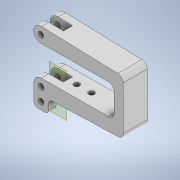
# Autodesk Inventor part: frame-1
Saved by Autodesk Inventor 2020 (Build 240168000, 168)
## iProperties
Created: 2019-10-15
Part Number: frame-1
Material: Generic
Document SubType Name: Modeling
Designer: psrob
Density: 1 g/cm^3
Appearance: Default
Author: psrob
Autodesk Inventor part; units mm, degrees
ref_plane "YZ Plane" through (0, 0, 0) normal (1, 0, 0) x (0, 1, 0)
ref_plane "XZ Plane" through (0, 0, 0) normal (0, 1, 0) x (-1, 0, 0)
ref_plane "XY Plane" through (0, 0, 0) normal (0, 0, 1) x (1, 0, 0)
sketch "Sketch1" plane through (0, 0, 0) normal (0, 0, 1) x (1, 0, 0)
  circle A0 centre (1.5, 0) radius 1.5
  circle A1 centre (1.648979, -24.25) radius 1.5
  circle A2 centre (1.648979, -31.25) radius 1.5
  circle A3 centre (1.5, 0) radius 4
  circle A4 centre (1.648979, -24.25) radius 4
  line L0 (1.5, 0) -> (33.5, 0)
  line L1 (1.648979, -24.25) -> (33.648979, -24.25)
  line L2 (33.5, 0) -> (33.648979, -24.25)
  line L3 (35.982292, 2.890075) -> (30.982386, 2.859359)
  line L4 (30.982386, 2.859359) -> (31.166687, -27.140075)
  line L5 (31.166687, -27.140075) -> (36.166593, -27.109359)
  line L6 (36.166593, -27.109359) -> (35.982292, 2.890075)
  line L7 (35.982292, 2.890075) -> (31.166687, -27.140075) construction
  line L8 (30.982386, 2.859359) -> (36.166593, -27.109359) construction
  line L9 (35.982292, 2.890075) -> (1.5, 4)
  line L10 (36.166593, -27.109359) -> (1.781342, -28.247809)
  line L11 (1.648979, -24.25) -> (1.781342, -28.247809)
  line L12 (1.516617, -20.252191) -> (31.123254, -20.070303)
  line L13 (1.5, 0) -> (1.524573, -3.999925)
  line L14 (1.524573, -3.999925) -> (31.023413, -3.818699)
  line L15 (1.5, 0) -> (1.5, 4)
  line L16 (5.648979, -24.25) -> (-2.351021, -24.25)
  line L17 (-2.351021, -24.25) -> (-2.351021, -35.25)
  line L18 (-2.351021, -35.25) -> (5.648979, -35.25)
  line L19 (5.648979, -35.25) -> (5.648979, -24.25)
  point P0 (0, 0)
  point P1 (33.57449, -12.125)
  point P2 (5.648979, -28.119757)
  point P3 (1.757239, 3.99172)
  point P4 (1.732213, -20.250866)
  dimension "d0" = 8
  dimension "d1" = 8
  dimension "d2" = 32
  dimension "d3" = 32
  dimension "d4" = 5
  dimension "d5" = 30
  dimension "d6" = 8
  dimension "d7" = 11
  constraints: 40 end point, 7 perpendicular, 5 point on circle, 4 parallel, 4 point on line, 3 horizontal, 3 midpoint, 2 centre point, 2 coincident, 1 horizontal alignment, 1 tangent, 1 vertical
  measures "d0" diameter of A3
  measures "d1" diameter of A4
  measures "d2" distance of L0.start L0.end
  measures "d3" distance of L1.start L1.end
  measures "d4" distance of L3.start L3.end
  measures "d5" distance of L4.end L3.end
  measures "d6" distance of L18.end L17.end
  measures "d7" distance of L17.end L16.end
extrude "Extrusion1" add sketch "Sketch1" along normal blind 4
sketch "Sketch2" plane through (0, 0, 4) normal (0, 0, 1) x (1, 0, 0)
  circle A0 centre (1.5, 0) radius 1.5
  circle A1 centre (1.648979, -24.25) radius 1.5
  point P0 (0, 0)
  constraints: 1 horizontal alignment
extrude "Extrusion2" cut sketch "Sketch2" against normal blind 5
fillet "Fillet1" radius 2 3 edges at (5.649, -28.1198, 2) (5.649, -35.25, 2) (-2.351, -35.25, 2)
fillet "Fillet2" radius 3 4 edges at (35.9823, 2.8901, 2) (36.1666, -27.1094, 2) (31.0234, -3.8187, 2) (31.1233, -20.0703, 2)
ref_plane "Work Plane1" through (-2.702041, -20.25, -5) normal (0, 0, -1) x (-1, 0, 0)
sketch "Sketch3" plane through (-2.702041, -20.25, -5) normal (0, 0, -1) x (-1, 0, 0)
  circle A0 centre (-4.351021, -4) radius 1.5
  circle A1 centre (-4.202041, 20.25) radius 1.5
  arc A2 (-38.850694, -3.939203) -> (-35.950022, -6.95599) centre (-35.850751, -3.957633) ccw
  line L0 (-10.284839, -7.805731) -> (-35.950022, -6.95599)
  arc A3 (-8.351021, -9.804635) -> (-10.284839, -7.805731) centre (-10.351021, -9.804635) ccw
  line L1 (-8.351021, -13) -> (-8.351021, -9.804635)
  arc A4 (-8.351021, -13) -> (-6.351021, -15) centre (-6.351021, -13) ccw
  line L2 (-2.351021, -15) -> (-6.351021, -15)
  arc A5 (-2.351021, -15) -> (-0.351021, -13) centre (-2.351021, -13) ccw
  line L3 (-0.351021, -4) -> (-0.351021, -13)
  arc A6 (-0.351021, -4) -> (-4.434254, -0.000866) centre (-4.351021, -4) ccw
  line L4 (-30.825352, 0.161267) -> (-4.434254, -0.000866)
  arc A7 (-33.806865, 3.179641) -> (-30.825352, 0.161267) centre (-30.806922, 3.161211) ccw
  line L5 (-33.743884, 13.431358) -> (-33.806865, 3.179641)
  arc A8 (-30.725511, 16.412871) -> (-33.743884, 13.431358) centre (-30.743941, 13.412928) ccw
  line L6 (-4.226615, 16.250075) -> (-30.725511, 16.412871)
  arc A9 (-4.226615, 16.250075) -> (-4.459281, 24.24172) centre (-4.202041, 20.25) ccw
  line L7 (-35.798641, 23.232961) -> (-4.459281, 24.24172)
  arc A10 (-35.798641, 23.232961) -> (-38.70207, 20.252944) centre (-35.702127, 20.234514) ccw
  line L8 (-38.850694, -3.939203) -> (-38.70207, 20.252944)
  circle A11 centre (-4.351021, -11) radius 1.5
  point P0 (-2.702041, 20.25)
extrude "Extrusion3" add sketch "Sketch3" along normal blind 4
sketch "Sketch4" plane through (0, 0, 0) normal (0, 0, -1) x (-1, 0, 0)
  arc A0 (-5.648979, -30.054635) -> (-7.582798, -28.055731) centre (-7.648979, -30.054635) ccw
  line L0 (-5.648979, -30.054635) -> (-5.648979, -33.25)
  arc A1 (-5.648979, -33.25) -> (-3.648979, -35.25) centre (-3.648979, -33.25) ccw
  line L1 (-3.648979, -35.25) -> (0.351021, -35.25)
  arc A2 (0.351021, -35.25) -> (2.351021, -33.25) centre (0.351021, -33.25) ccw
  line L2 (2.351021, -33.25) -> (2.351021, -24.25)
  arc A3 (2.351021, -24.25) -> (-1.732213, -20.250866) centre (-1.648979, -24.25) ccw
  line L3 (-1.732213, -20.250866) -> (-28.123311, -20.088733)
  arc A4 (-31.104824, -17.070359) -> (-28.123311, -20.088733) centre (-28.104881, -17.088789) ccw
  line L4 (-31.104824, -17.070359) -> (-31.041843, -6.818642)
  arc A5 (-28.02347, -3.837129) -> (-31.041843, -6.818642) centre (-28.0419, -6.837072) ccw
  line L5 (-28.02347, -3.837129) -> (-1.524573, -3.999925)
  arc A6 (-1.524573, -3.999925) -> (-1.757239, 3.99172) centre (-1.5, 0) ccw
  line L6 (-1.757239, 3.99172) -> (-33.0966, 2.982961)
  arc A7 (-33.0966, 2.982961) -> (-36.000029, 0.002944) centre (-33.000086, -0.015486) ccw
  line L7 (-36.000029, 0.002944) -> (-36.148653, -24.189203)
  arc A8 (-36.148653, -24.189203) -> (-33.247981, -27.20599) centre (-33.14871, -24.207633) ccw
  line L8 (-33.247981, -27.20599) -> (-7.582798, -28.055731)
  circle A9 centre (-1.648979, -31.25) radius 1.5
  circle A10 centre (-1.5, 0) radius 1.5
  circle A11 centre (-1.648979, -24.25) radius 1.5
  line L9 (-33.247981, -27.20599) -> (-7.582798, -28.055731)
  line L10 (-7.582798, -28.055731) -> (-7.582798, -20.214923)
  line L11 (-28.123311, -20.088733) -> (-1.732213, -20.250866)
  line L12 (-28.02347, -3.837129) -> (-1.524573, -3.999925)
  line L13 (-7.582798, -3.962706) -> (-7.582798, 3.804205)
  line L14 (-1.757239, 3.99172) -> (-33.0966, 2.982961)
  point P0 (0, 0)
  point P1 (-7.582798, 3.804205)
  constraints: 5 point on line, 4 end point, 1 vertical
extrude "Extrusion4" add sketch "Sketch4" along normal blind 5 contours L8 A8 L7 A7 L6 L13 L5 A5 L4 A4 L3 L10
chamfer "Chamfer1" distance 2 angle 45 4 edges at (7.5828, -20.2149, -2.5) (7.5828, -28.0557, -2.5) (7.5828, 3.8042, -2.5) (7.5828, -3.9627, -2.5)
sketch "Sketch8" plane through (7.582798, -28.055731, 0) normal (0.0330906, -0.9994524, 0) x (0.9994524, 0.0330906, 0)
  line L0 (0, -5) -> (2, -5)
  line L1 (0, -5) -> (0, -9)
  line L2 (25.679246, -9) -> (0, -9)
  line L3 (25.679246, 4) -> (25.679246, -9)
  line L4 (0, 4) -> (25.679246, 4)
  line L5 (0, 0) -> (0, 4)
  line L6 (2, 0) -> (0, 0)
  line L7 (2, -5) -> (2, 0)
  line L8 (2, -2.5) -> (7, -2.5)
  line L9 (7, -2.5) -> (15, -2.5)
  circle A0 centre (7, -2.5) radius 1.5
  circle A1 centre (15, -2.5) radius 1.5
  point P0 (-6.650266, 0)
  dimension "d39" = 5
  dimension "d40" = 8
  dimension "d41" = 3
  dimension "d42" = 3
  constraints: 4 end point, 2 centre point, 2 coincident, 1 horizontal, 1 midpoint, 1 point on line
  measures "d39" distance of L8.start L8.end
  measures "d40" distance of L8.end L9.end
  measures "d41" diameter of A0
  measures "d42" diameter of A1
extrude "Extrusion8" cut sketch "Sketch8" against normal blind 10 contours A0 L9 L8 | L8 L9 A0 | A1
thicken "Thicken1" operation add thickness 10 both sides no extend neighbours yes toward (0.9999811, 0.0061434, 0) faces at (36.04957, -8.061105, -0.333333)
thicken "Thicken2" operation add thickness 10 both sides no extend neighbours yes toward (0.9999811, 0.0061434, 0) faces at (31.083831, -13.65312, -0.333333)
body "Solid1"
